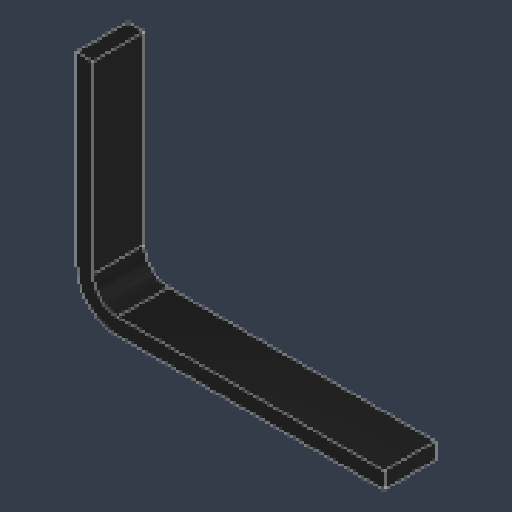
# Autodesk Inventor part: Corner
Saved by Autodesk Inventor 2023.4 (Build 274418000, 418)
## iProperties
Created: 2024-02-24
Part Number: Corner
Material: Generic
Document SubType Name: Modeling
Designer: JoaoSilva
Density: 1 g/cm^3
Appearance: Smooth - Black
Author: JoaoSilva
Autodesk Inventor part; units mm, degrees
ref_plane "YZ Plane" through (0, 0, 0) normal (1, 0, 0) x (0, 1, 0)
ref_plane "XZ Plane" through (0, 0, 0) normal (0, 1, 0) x (-1, 0, 0)
ref_plane "XY Plane" through (0, 0, 0) normal (0, 0, 1) x (1, 0, 0)
sketch "Sketch1" plane through (0, 0, 0) normal (0, 0, 1) x (1, 0, 0)
  line L0 (-74.8, 54.8) -> (74.8, 54.8)
  line L1 (74.8, 54.8) -> (74.8, -54.8)
  line L2 (74.8, -54.8) -> (-74.8, -54.8)
  line L3 (-74.8, -54.8) -> (-74.8, 54.8)
  line L4 (-74.8, 54.8) -> (74.8, -54.8) construction
  line L5 (74.8, 54.8) -> (-74.8, -54.8) construction
  line L6 (-66.8, 54.8) -> (-66.8, -46.8)
  line L7 (-66.8, -46.8) -> (74.8, -46.8)
  point P0 (0, 0)
  dimension "d0" = 149.6
  dimension "d1" = 109.6
  dimension "d2" = 8
  dimension "d3" = 8
  constraints: 16 end point, 3 perpendicular, 2 midpoint, 2 parallel, 2 point on line, 1 horizontal
  measures "d0" distance of L1.end L2.end
  measures "d1" distance of L2.end L0.start
  measures "d2" distance between parallel lines of L2 L7
  measures "d3" distance between parallel lines of L3 L6
extrude "Extrusion1" add sketch "Sketch1" along normal blind 25 contours L0 L6 L7 L1 L2 L3
fillet "Fillet1" radius 12 1 edges at (-66.8, -46.8, 12.5)
fillet "Fillet2" radius 20 1 edges at (-74.8, -54.8, 12.5)
sketch "Sketch2" plane through (0, 0, 25) normal (0, 0, 1) x (1, 0, 0)
  circle A0 centre (25.2, -44.8) radius 5
  circle A1 centre (-60.8, -40.8) radius 5
  circle A2 centre (-64.8, 18.2) radius 5
  line L0 (-54.8, -54.8) -> (74.8, -54.8) projected
  line L1 (-74.8, 54.8) -> (-74.8, -34.8) projected
  point P0 (0, 0)
  dimension "d8" = 10
  dimension "d9" = 10
  dimension "d10" = 14
  dimension "d11" = 14
  dimension "d12" = 73
  dimension "d13" = 100
  dimension "d14" = 10
  constraints: 3 centre point, 2 equal radius
  measures "d8" distance from line of L0 A0.centre
  measures "d9" distance from line of L1 A2.centre
  measures "d10" distance from line of L0 A1.centre
  measures "d11" distance from line of L1 A1.centre
  measures "d12" distance from line of L0 A2.centre
  measures "d13" distance from line of A0.centre L1
  measures "d14" diameter of A0
extrude "Extrusion2" add sketch "Sketch2" against normal up to surface (25 mm away)
sketch "Sketch3" plane through (0, 0, 25) normal (0, 0, 1) x (1, 0, 0)
  arc A0 (-66.8, 13.6174) -> (-66.8, 22.7826) centre (-64.8, 18.2) ccw projected
  arc A1 (-59.8147, -45.702) -> (-65.702, -39.8147) centre (-60.8, -40.8) ccw projected
  arc A2 (29.7826, -46.8) -> (20.6174, -46.8) centre (25.2, -44.8) ccw projected
  point P0 (0, 0)
hole "Hole1" at (-64.8, 18.2, 25) at (-60.8, -40.8, 25) at (25.2, -44.8, 25) direction (0, 0, -1) diameter 5.6 depth 15
fillet "Fillet3" radius 5 6 edges at (20.6174, -46.8, 12.5) (29.7826, -46.8, 12.5) (-59.8147, -45.702, 12.5) (-65.702, -39.8147, 12.5) (-66.8, 13.6174, 12.5) (-66.8, 22.7826, 12.5)
fillet "Fillet4" radius 0.4 4 edges at (-74.8, 54.8, 12.5) (-66.8, 54.8, 12.5) (74.8, -54.8, 12.5) (74.8, -46.8, 12.5)
equation "\"d3\" = d2"
equation "\"d9\" = d8"
equation "\"d11\" = d10"
body "Solid1"
